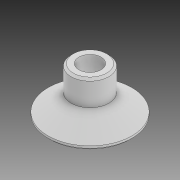
# Autodesk Inventor part: SingleWheelPost
Saved by Autodesk Inventor 2020 (Build 240168000, 168)
## iProperties
Created: 2020-11-03
Part Number: SingleWheelPost
Material: Generic
Document SubType Name: Modeling
Designer: DDeGo
Density: 1 g/cm^3
Appearance: Default
Author: DDeGo
Autodesk Inventor part; units mm, degrees
ref_plane "YZ Plane" through (0, 0, 0) normal (1, 0, 0) x (0, 1, 0)
ref_plane "XZ Plane" through (0, 0, 0) normal (0, 1, 0) x (-1, 0, 0)
ref_plane "XY Plane" through (0, 0, 0) normal (0, 0, 1) x (1, 0, 0)
sketch "Sketch1" plane through (0, 0, 0) normal (1, 0, 0) x (0, 1, 0)
  line L0 (0, 0) -> (11, 0) construction
  line L1 (11, 0) -> (11, -2.65) construction
  line L2 (11, -2.65) -> (0, -2.65)
  line L3 (0, -2.65) -> (0, 0) construction
  line L4 (11, -2.65) -> (11, -4.5)
  line L5 (11, -4.5) -> (5, -4.5)
  line L6 (5, -4.5) -> (1, -10)
  line L7 (1, -10) -> (0, -10)
  line L8 (0, -10) -> (0, -2.65)
  dimension "d0" = 1
  dimension "d1" = 6
  dimension "d2" = 2.65
  dimension "d3" = 4.5
  dimension "d4" = 5
  dimension "d5" = 10
  constraints: 18 end point, 4 perpendicular, 2 vertical, 1 horizontal, 1 parallel
  measures "d0" distance of L6.end L7.end
  measures "d1" distance of L4.end L5.end
  measures "d2" distance between parallel lines of L0 L2
  measures "d3" distance between parallel lines of L0 L5
  measures "d4" distance from line of L8 L5.end
  measures "d5" distance between parallel lines of L7 L0
revolve "Revolution1" add sketch "Sketch1" angle 360 about axis through (0, 0, 0) along (0, 1, 0)
chamfer "Chamfer1" distance 0.5 angle 45 2 edges at (0, 11, 4.5) (0, 0, 10)
body "Solid1"
